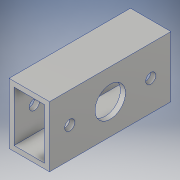
# Autodesk Inventor part: 2AM-17-P-5209 - cylinder mount
Saved by Autodesk Inventor 2017 (Build 210142000, 142)
## iProperties
Created: 2017-09-30
Part Number: 2AM-17-P-5209 - cylinder mount
Material: Aluminum 6061
Document SubType Name: Modeling
Designer: Gus
Density: 2.7 g/cm^3
Appearance: Aluminum - Flat
Mass: 90.2705 g
Surface Area: 223.851 cm^2
Volume: 33.4335 cm^3
Author: Gus
Autodesk Inventor part; units mm, degrees
ref_plane "YZ Plane" through (0, 0, 0) normal (1, 0, 0) x (0, 1, 0)
ref_plane "XZ Plane" through (0, 0, 0) normal (0, 1, 0) x (-1, 0, 0)
ref_plane "XY Plane" through (0, 0, 0) normal (0, 0, 1) x (1, 0, 0)
sketch "Sketch1" plane through (0, 0, 0) normal (0, 0, 1) x (1, 0, 0)
  line L0 (-12.7, -19.05) -> (12.7, -19.05)
  line L1 (12.7, -19.05) -> (12.7, 19.05)
  line L2 (12.7, 19.05) -> (-12.7, 19.05)
  line L3 (-12.7, 19.05) -> (-12.7, -19.05)
  line L4 (-12.7, -19.05) -> (12.7, 19.05) construction
  line L5 (12.7, -19.05) -> (-12.7, 19.05) construction
  line L6 (-9.525, 15.875) -> (9.525, 15.875)
  line L7 (9.525, 15.875) -> (9.525, -15.875)
  line L8 (9.525, -15.875) -> (-9.525, -15.875)
  line L9 (-9.525, -15.875) -> (-9.525, 15.875)
  point P0 (0, 0)
  dimension "d0" = 25.4
  dimension "d1" = 38.1
  dimension "d2" = 3.175
  constraints: 20 end point, 4 parallel, 2 midpoint, 2 perpendicular, 1 horizontal, 3 other
  measures "d0" distance of L2.end L1.end
  measures "d1" distance of L1.end L0.end
  measures "d2" distance between parallel lines of L2 L6
extrude "Extrusion1" add sketch "Sketch1" along normal mid plane 127
sketch "Sketch2" plane through (12.7, -19.05, 63.5) normal (1, 0, 0) x (0, 0, -1)
  circle A0 centre (63.5, 19.05) radius 3.175
  dimension "d5" = 6.35
  constraints: 1 centre point, 1 coincident
  measures "d5" diameter of A0
extrude "Extrusion2" cut sketch "Sketch2" against normal through all
pattern_linear "Rectangular Pattern1" count 4 spacing 25.4 along (0, 0, 1) of "Extrusion2" first direction both ways yes skipped copies 4
hole "Hole1" at (12.7, 0, 0) direction (-1, 0, 0) diameter 15.875 end through all
hole "Hole2" at (12.7, 0, 0) direction (-1, 0, 0) diameter 19.05 end through all
sketch "Sketch3" plane through (12.7, -19.05, 63.5) normal (1, 0, 0) x (0, 0, -1)
  line L0 (127, 38.1) -> (0, 38.1) projected
  line L1 (63.5, 38.1) -> (63.5, 0)
  line L2 (0, 0) -> (127, 0) projected
  line L3 (25.4, 38.1) -> (25.4, 0)
  line L4 (0, 0) -> (0, 38.1) projected
  line L5 (101.6, 38.1) -> (101.6, 0)
  line L6 (127, 38.1) -> (127, 0) projected
  point P0 (63.5, 19.05)
  dimension "d29" = 25.4
  dimension "d30" = 25.4
  constraints: 6 end point, 4 point on line, 2 midpoint, 2 perpendicular
  measures "d29" distance between parallel lines of L4 L3
  measures "d30" distance between parallel lines of L6 L5
split body "Split1" sketch "Sketch3" result one side removed curves L3 removed pieces at (-12.2, -6.35, 46.5667)
split body "Split2" sketch "Sketch3" result one side removed curves L5 removed pieces at (12.2, -6.35, -55.0333)
body "Solid1"
